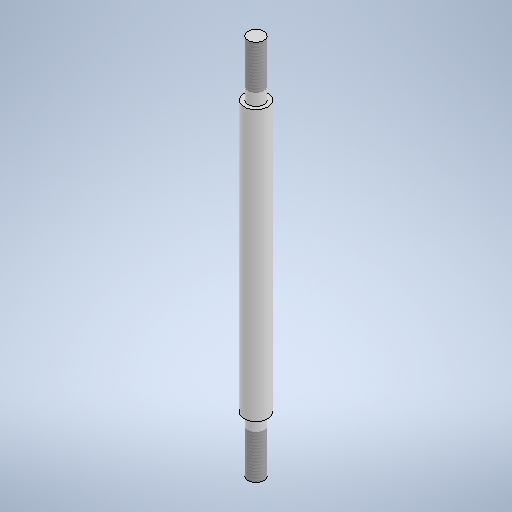
# Autodesk Inventor part: 1018
Saved by Autodesk Inventor 2025 (Build 290162010, 162A)
## iProperties
Created: 2024-07-12
Part Number: 1018
Material: Generisch
Document SubType Name: Modeling
Designer: ffogue
Density: 1 g/cm^3
Appearance: Vorgabe
Author: ffogue
Autodesk Inventor part; units mm, degrees
ref_plane "YZ Plane" through (0, 0, 0) normal (1, 0, 0) x (0, 1, 0)
ref_plane "XZ Plane" through (0, 0, 0) normal (0, 1, 0) x (-1, 0, 0)
ref_plane "XY Plane" through (0, 0, 0) normal (0, 0, 1) x (1, 0, 0)
sketch "Skizze1" plane through (0, 0, 0) normal (0, 1, 0) x (-1, 0, 0)
  line L0 (0, 0) -> (2, 0)
  line L1 (2, 0) -> (2, -14)
  line L2 (2, -14) -> (3, -14)
  line L3 (3, -14) -> (3, -82)
  line L4 (3, -82) -> (2, -82)
  line L5 (2, -82) -> (2, -96)
  line L6 (2, -96) -> (0, -96)
  line L7 (0, -96) -> (0, 0)
  point P0 (1, -96)
  dimension "d0" = 96
  dimension "d1" = 68
  dimension "d2" = 14
  dimension "d3" = 4
  dimension "d4" = 6
  constraints: 16 end point, 5 perpendicular, 2 point on line, 1 horizontal, 1 midpoint, 1 vertical alignment
  measures "d0" distance of L6.end L0.start
  measures "d1" distance of L2.end L3.end
  measures "d2" distance from line of point (1, -96) L4
  measures "d3" diameter of L5 L7
  measures "d4" diameter of L3 L7
revolve "Umdrehung1" add sketch "Skizze1" angle 360 about axis through (0, 0, -96) along (0, 0, 1)
thread "Gewinde1" size "M4x0.7" class "6g" standard "ISO Metric profile" length 11
thread "Gewinde2" size "M4x0.7" class "6g" standard "ISO Metric profile" length 11
